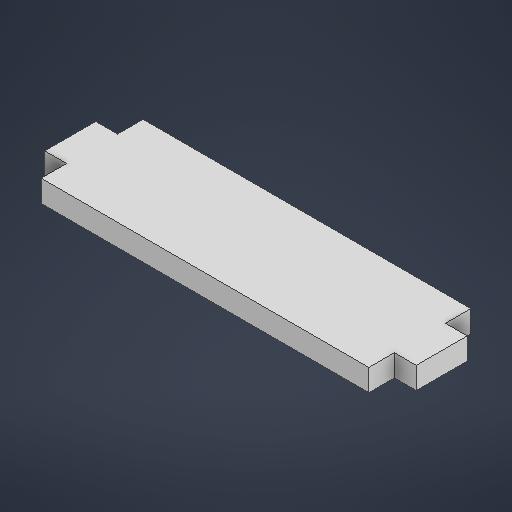
# Autodesk Inventor part: Spojka
Saved by Autodesk Inventor 2026 (Build 300175000, 175)
## iProperties
Created: 2025-06-20
Part Number: Spojka
Material: Všeobecné
Document SubType Name: Modeling
Designer: vadim
Density: 1 g/cm^3
Appearance: Výchozí
Author: vadim
Autodesk Inventor part; units mm, degrees
ref_plane "YZ Plane" through (0, 0, 0) normal (1, 0, 0) x (0, 1, 0)
ref_plane "XZ Plane" through (0, 0, 0) normal (0, 1, 0) x (-1, 0, 0)
ref_plane "XY Plane" through (0, 0, 0) normal (0, 0, 1) x (1, 0, 0)
sketch "Náčrt1" plane through (0, 0, 0) normal (0, 1, 0) x (-1, 0, 0)
  line L0 (22.5, 7) -> (-22.5, 7)
  line L1 (-22.5, -7) -> (22.5, -7)
  line L2 (22.5, 7) -> (-22.5, -7) construction
  line L3 (-22.5, 7) -> (22.5, -7) construction
  line L4 (25.5, -3.5) -> (22.5, -3.5)
  line L5 (22.5, 0) -> (22.5, 3.5)
  line L6 (22.5, 3.5) -> (25.5, 3.5)
  line L7 (25.5, 3.5) -> (25.5, -3.5)
  line L8 (25.5, -3.5) -> (22.5, 3.5) construction
  line L9 (22.5, -3.5) -> (25.5, 3.5) construction
  line L10 (22.5, 0) -> (-22.5, 0)
  line L11 (-22.5, 3.5) -> (-25.5, 3.5)
  line L12 (-25.5, 3.5) -> (-25.5, -3.5)
  line L13 (-25.5, -3.5) -> (-22.5, -3.5)
  line L14 (-22.5, 3.5) -> (-25.5, -3.5) construction
  line L15 (-25.5, 3.5) -> (-22.5, -3.5) construction
  line L16 (-22.5, 7) -> (-22.5, 3.5)
  line L17 (-22.5, -3.5) -> (-22.5, -7)
  line L18 (22.5, -7) -> (22.5, -3.5)
  line L19 (22.5, 0) -> (22.5, 7)
  point P0 (0, 0)
  point P1 (24, 0)
  point P2 (-24, 0)
  point P3 (22.5, -5.25)
  dimension "d0" = 14
  dimension "d2" = 7
  dimension "d5" = 7
  dimension "d8" = 3
  dimension "d9" = 3
  dimension "d12" = 45
  constraints: 40 end point, 8 parallel, 7 midpoint, 4 perpendicular, 3 horizontal, 2 collinear, 1 point on line, 1 other
  measures "d0" distance of L1.start L0.end
  measures "d2" distance of L5.end L4.end
  measures "d5" distance of L12.end L11.end
  measures "d8" distance between parallel lines of L19 L7
  measures "d9" distance between parallel lines of L17 L12
  measures "d12" distance from line of L17 point (22.5, -5.25)
extrude "Vysunutí1" add sketch "Náčrt1" along normal blind 3
